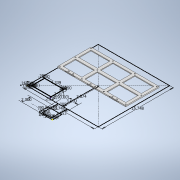
# Autodesk Inventor part: WellPlateFrame - 3L - Part1
Saved by Autodesk Inventor 2020 (Build 240168000, 168)
## iProperties
Created: 2023-02-18
Part Number: WellPlateFrame - 3L - Part1
Material: Generic
Document SubType Name: Modeling
Designer: Beaucage
Density: 1 g/cm^3
Appearance: Default
Author: Beaucage
Autodesk Inventor part; units mm, degrees
ref_plane "YZ Plane" through (0, 0, 0) normal (1, 0, 0) x (0, 1, 0)
ref_plane "XZ Plane" through (0, 0, 0) normal (0, 1, 0) x (-1, 0, 0)
ref_plane "XY Plane" through (0, 0, 0) normal (0, 0, 1) x (1, 0, 0)
sketch "Sketch1" plane through (0, 0, 0) normal (0, 1, 0) x (-1, 0, 0)
  line L0 (0, 0) -> (76.2, 0)
  line L1 (76.2, 0) -> (76.2, -50.8)
  line L2 (76.2, -50.8) -> (0, -50.8)
  line L3 (0, -50.8) -> (0, 0)
  line L4 (38.1, 0) -> (38.1, -6.35)
  line L5 (38.1, -6.35) -> (12.7, -6.35)
  line L6 (38.1, -6.35) -> (63.5, -6.35)
  line L7 (38.1, -6.35) -> (63.5, -6.35) construction
  line L8 (63.5, -6.35) -> (63.5, -19.05)
  line L9 (12.7, -6.35) -> (12.7, -19.05)
  line L10 (63.5, -19.05) -> (63.5, -25.4)
  line L11 (12.7, -19.05) -> (12.7, -25.4)
  line L12 (63.5, -19.05) -> (63.5, -94.05)
  line L13 (63.5, -19.05) -> (138.5, -19.05) construction
  line L14 (12.7, -19.05) -> (12.7, -94.05)
  line L15 (63.5, -94.05) -> (38.1, -94.05)
  line L16 (38.1, -94.05) -> (38.1, -294.05)
  line L17 (38.1, -94.05) -> (238.1, -94.05) construction
  line L18 (238.1, -494.05) -> (-161.9, -494.05)
  line L19 (-161.9, -494.05) -> (-161.9, -94.05)
  line L20 (-161.9, -94.05) -> (238.1, -94.05)
  line L21 (238.1, -94.05) -> (238.1, -494.05)
  line L22 (238.1, -494.05) -> (-161.9, -94.05) construction
  line L23 (-161.9, -494.05) -> (238.1, -94.05) construction
  point P0 (63.5, -50.8)
  point P1 (12.7, -50.8)
  dimension "d0" = 76.2
  dimension "d1" = 50.8
  dimension "d2" = 6.35
  dimension "d3" = 25.4
  dimension "d4" = 25.4
  dimension "d5" = 0
  dimension "d6" = 12.7
  dimension "d7" = 12.7
  dimension "d8" = 6.35
  dimension "d9" = 6.35
  dimension "d10" = 75
  dimension "d11" = 90
  dimension "d12" = 75
  dimension "d13" = 25.4
  dimension "d14" = 200
  dimension "d15" = 90
  dimension "d16" = 400
  dimension "d17" = 400
  constraints: 48 end point, 7 horizontal, 6 vertical, 4 parallel, 4 perpendicular, 3 equal length, 3 midpoint, 1 point on line
  measures "d0" distance of L1.end L2.end
  measures "d1" distance of L0.end L1.end
  measures "d2" distance of L4.start L4.end
  measures "d3" distance of L4.end L5.end
  measures "d4" distance of L4.end L6.end
  measures "d5" distance between parallel lines of L6 L7
  measures "d6" distance of L6.end L8.end
  measures "d7" distance of L5.end L9.end
  measures "d8" distance of L8.end L10.end
  measures "d9" distance of L9.end L11.end
  measures "d10" distance of L8.end L12.end
  measures "d11" angle of L12 L13
  measures "d12" distance of L9.end L14.end
  measures "d13" distance of L12.end L15.end
  measures "d14" distance of L15.end L16.end
  measures "d15" angle of L16 L17
  measures "d16" distance of L19.end L20.end
  measures "d17" distance of L18.end L19.end
extrude "Extrusion1" add sketch "Sketch1" along normal blind 6.35
hole "Hole1" at (-12.7, 0, -6.35) at (-12.7, 0, -19.05) at (-63.5, 0, -6.35) at (-63.5, 0, -19.05) direction (0, 1, 0) diameter 6.604 end through all
sketch "Sketch2" plane through (0, 0, 0) normal (0, -1, 0) x (1, 0, 0)
  line L0 (-238.1, -94.05) -> (-63.5, -94.05) projected
  line L1 (-238.1, -94.05) -> (-238.1, -100.4)
  line L2 (-238.1, -94.05) -> (-231.75, -94.05) construction
  line L3 (-238.1, -100.4) -> (-231.75, -100.4)
  line L4 (-231.75, -100.4) -> (-225.4, -100.4)
  line L5 (-225.4, -100.4) -> (-225.4, -106.75)
  line L6 (-225.4, -106.75) -> (-115.2, -106.75)
  line L7 (-115.2, -106.75) -> (-115.2, -180.75)
  line L8 (-115.2, -180.75) -> (-225.4, -180.75)
  line L9 (-225.4, -180.75) -> (-225.4, -106.75)
  line L10 (-115.2, -106.75) -> (-115.2, -100.4)
  line L11 (-115.2, -100.4) -> (-108.85, -100.4)
  line L12 (-225.4, -180.75) -> (-231.75, -180.75)
  line L13 (-231.75, -180.75) -> (-231.75, -187.1)
  line L14 (-115.2, -180.75) -> (-115.2, -187.1)
  line L15 (-115.2, -187.1) -> (-108.85, -187.1)
  line L16 (-225.4, -106.75) -> (-225.4, -114.75)
  line L17 (-225.4, -106.75) -> (-217.4, -106.75) construction
  line L18 (-225.4, -106.75) -> (-223.4, -106.75)
  line L19 (-223.4, -106.75) -> (-223.4, -108.75)
  line L20 (-223.4, -108.75) -> (-225.4, -108.75)
  line L21 (-225.4, -108.75) -> (-225.4, -106.75)
  line L22 (-115.2, -180.75) -> (-117.2, -180.75)
  line L23 (-117.2, -180.75) -> (-117.2, -178.75)
  line L24 (-117.2, -178.75) -> (-115.2, -178.75)
  line L25 (-115.2, -178.75) -> (-115.2, -180.75)
  line L26 (-223.4, -108.75) -> (-117.2, -108.75)
  line L27 (-117.2, -108.75) -> (-117.2, -178.75)
  line L28 (-117.2, -178.75) -> (-223.4, -178.75)
  line L29 (-223.4, -178.75) -> (-223.4, -108.75)
  point P0 (0, 0)
  dimension "d27" = 6.35
  dimension "d28" = 90
  dimension "d29" = 6.35
  dimension "d30" = 6.35
  dimension "d31" = 6.35
  dimension "d32" = 110.2
  dimension "d33" = 74
  dimension "d34" = 6.35
  dimension "d35" = 6.35
  dimension "d36" = 6.35
  dimension "d37" = 6.35
  dimension "d38" = 6.35
  dimension "d39" = 8
  dimension "d40" = 90
  dimension "d41" = 2
  dimension "d42" = 2
  dimension "d43" = 2
  dimension "d44" = 2
  constraints: 58 end point, 11 perpendicular, 8 horizontal, 8 parallel, 4 vertical
  measures "d27" distance of L0.start L1.end
  measures "d28" angle of L1 L2
  measures "d29" distance of L1.end L3.end
  measures "d30" distance of L3.end L4.end
  measures "d31" distance of L4.end L5.end
  measures "d32" distance of L7.end L8.end
  measures "d33" distance of L6.end L7.end
  measures "d34" distance of L10.end L11.end
  measures "d35" distance of L8.end L12.end
  measures "d36" distance of L12.end L13.end
  measures "d37" distance of L7.end L14.end
  measures "d38" distance of L14.end L15.end
  measures "d39" distance of L5.end L16.end
  measures "d40" angle of L16 L17
  measures "d41" distance of L19.end L20.end
  measures "d42" distance of L18.end L19.end
  measures "d43" distance of L23.end L24.end
  measures "d44" distance of L22.end L23.end
extrude "Extrusion2" cut sketch "Sketch2" against normal through all contours L26 L27 L28 L29
hole "Hole2" at (-231.75, 0, -100.4) at (-231.75, 0, -187.1) at (-108.85, 0, -100.4) at (-108.85, 0, -187.1) direction (0, 1, 0) diameter 5.1562 end through all
extrude "Extrusion3" cut sketch "Sketch2" against normal blind 2 contours L6 L19 L20 L9 | L6 L7 L24 L27 L26 L19 | L20 L29 L28 L23 L8 L9 | L7 L8 L23 L24
pattern_linear "Rectangular Pattern1" count 3 spacing 122.9106 along (1, 0, 0) count 4 spacing 86.9442 along (0, 0, -1) of "Extrusion2", "Hole2", "Extrusion3"
sketch "Sketch3" plane through (0, 0, 0) normal (0, -1, 0) x (1, 0, 0)
  circle A0 centre (136.9712, -447.9326) radius 2.5781 projected
  line L0 (136.9712, -447.9326) -> (143.3212, -447.9326)
  line L1 (143.3212, -447.9326) -> (143.3212, -454.2826)
  line L2 (143.3212, -454.2826) -> (136.9712, -454.2826)
  line L3 (136.9712, -454.2826) -> (136.9712, -447.9326)
  line L4 (-12.7, -94.05) -> (161.9, -94.05) projected
  line L5 (143.3212, -454.2826) -> (161.9, -454.2826)
  line L6 (161.9, -454.2826) -> (161.9, -94.05)
  line L7 (161.9, -94.05) -> (143.3212, -94.05)
  line L8 (143.3212, -94.05) -> (143.3212, -454.2826)
  line L9 (161.9, -454.2826) -> (-238.1, -454.2826)
  line L10 (-238.1, -454.2826) -> (-238.1, -500.3541)
  line L11 (-238.1, -500.3541) -> (161.9, -500.3541)
  line L12 (161.9, -500.3541) -> (161.9, -454.2826)
  point P0 (0, 0)
  dimension "d62" = 6.35
  dimension "d63" = 6.35
  constraints: 24 end point, 6 parallel, 3 horizontal, 3 perpendicular
  measures "d62" distance of L1.end L2.end
  measures "d63" distance of L0.end L1.end
extrude "Extrusion4" cut sketch "Sketch3" against normal through all contours L8 L4 L6 L5 L1 | L2 L5 L12 L11 L10 L9
sketch "Sketch4" plane through (0, 6.35, 0) normal (0, 1, 0) x (1, 0, 0)
  line L0 (-238.1, 454.2826) -> (-238.1, 94.05) projected
  line L1 (143.3212, 94.05) -> (143.3212, 454.2826) projected
  line L2 (-238.1, 454.2826) -> (143.3212, 454.2826)
  line L3 (143.3212, 454.2826) -> (143.3212, 265.3699)
  line L4 (143.3212, 265.3699) -> (-238.1, 265.3699)
  line L5 (-238.1, 265.3699) -> (-238.1, 454.2826)
  line L6 (143.3212, 265.3699) -> (-238.1, 265.3699)
  line L7 (-238.1, 265.3699) -> (-238.1, 0)
  line L8 (-238.1, 0) -> (143.3212, 0)
  line L9 (143.3212, 0) -> (143.3212, 265.3699)
  line L10 (-223.1708, 265.3699) -> (-238.1, 265.3699)
  line L11 (-117.2, 265.6942) -> (-223.4, 265.6942) projected
  line L12 (-223.4, 265.6942) -> (-238.1, 265.6942)
  line L13 (-238.1, 265.6942) -> (143.3212, 265.6942)
  line L14 (143.3212, 265.6942) -> (143.3212, 0)
  line L15 (143.3212, 0) -> (-238.1, 0)
  line L16 (-238.1, 0) -> (-238.1, 265.6942)
  line L17 (-225.4, 267.6942) -> (-238.1, 267.6942)
  line L18 (-238.1, 454.2826) -> (-238.1, 94.05) projected
  line L19 (-238.1, 267.6942) -> (143.3212, 267.6942)
  line L20 (143.3212, 267.6942) -> (143.3212, 0)
  line L21 (143.3212, 0) -> (-238.1, 0)
  line L22 (-238.1, 0) -> (-238.1, 267.6942)
  point P0 (0, 0)
  point P1 (143.3212, 265.6942)
  point P2 (143.3212, 267.6942)
  constraints: 38 end point, 8 parallel, 5 horizontal, 5 perpendicular, 5 point on line, 1 collinear
extrude "Extrusion5" cut sketch "Sketch4" against normal blind 25.4 contours L17 L19 L1 L13 L11 L12 L0 | L12 L11 L13 L1 L4 L0 | L4 L1 L9 L8 L7 L0
sketch "Sketch5" plane through (-238.1, 0, -267.6942) normal (0, 0, 1) x (1, 0, 0)
  line L0 (120.9, 2) -> (14.7, 2) projected
  line L1 (243.8106, 2) -> (137.6106, 2) projected
  line L2 (366.7212, 2) -> (260.5212, 2) projected
  line L3 (120.9, 6.35) -> (14.7, 6.35) projected
  line L4 (67.8, 6.35) -> (67.8, 3.175)
  line L5 (42.4, 4.7625) -> (93.2, 4.7625)
  line L6 (93.2, 4.7625) -> (93.2, 1.5875)
  line L7 (93.2, 1.5875) -> (42.4, 1.5875)
  line L8 (42.4, 1.5875) -> (42.4, 4.7625)
  line L9 (42.4, 4.7625) -> (93.2, 1.5875) construction
  line L10 (93.2, 4.7625) -> (42.4, 1.5875) construction
  line L11 (381.4212, 6.35) -> (0, 6.35) projected
  line L12 (190.7106, 6.35) -> (190.7106, 3.175)
  line L13 (165.3106, 1.5875) -> (216.1106, 1.5875)
  line L14 (216.1106, 1.5875) -> (216.1106, 4.7625)
  line L15 (216.1106, 4.7625) -> (165.3106, 4.7625)
  line L16 (165.3106, 4.7625) -> (165.3106, 1.5875)
  line L17 (165.3106, 1.5875) -> (216.1106, 4.7625) construction
  line L18 (216.1106, 1.5875) -> (165.3106, 4.7625) construction
  line L19 (260.5212, 6.35) -> (366.7212, 6.35) projected
  line L20 (313.6212, 6.35) -> (313.6212, 3.175)
  line L21 (288.2212, 1.5875) -> (339.0212, 1.5875)
  line L22 (339.0212, 1.5875) -> (339.0212, 4.7625)
  line L23 (339.0212, 4.7625) -> (288.2212, 4.7625)
  line L24 (288.2212, 4.7625) -> (288.2212, 1.5875)
  line L25 (288.2212, 1.5875) -> (339.0212, 4.7625) construction
  line L26 (339.0212, 1.5875) -> (288.2212, 4.7625) construction
  point P0 (238.1, 0)
  dimension "d68" = 3.175
  dimension "d69" = 50.8
  dimension "d70" = 3.175
  dimension "d71" = 50.8
  dimension "d72" = 3.175
  dimension "d73" = 3.175
  dimension "d74" = 50.8
  constraints: 42 end point, 9 midpoint, 6 parallel, 3 horizontal, 3 perpendicular, 3 vertical
  measures "d68" distance of L4.start L4.end
  measures "d69" distance of L6.end L7.end
  measures "d70" distance of L5.end L6.end
  measures "d71" distance of L15.end L14.end
  measures "d72" distance of L14.end L13.end
  measures "d73" distance of L20.start L20.end
  measures "d74" distance of L23.end L22.end
extrude "Extrusion6" cut sketch "Sketch5" against normal blind 3.175
sketch "Sketch6" plane through (0, 6.35, 0) normal (0, 1, 0) x (1, 0, 0)
  line L0 (-195.7, 267.6942) -> (-144.9, 267.6942) projected
  line L1 (-72.7894, 267.6942) -> (-21.9894, 267.6942) projected
  line L2 (50.1212, 267.6942) -> (100.9212, 267.6942) projected
  line L3 (-170.3, 267.6942) -> (-170.3, 274.0442)
  line L4 (-170.3, 274.0442) -> (-157.6, 274.0442)
  line L5 (-157.6, 274.0442) -> (-183, 274.0442)
  line L6 (-238.1, 267.6942) -> (143.3212, 267.6942) projected
  line L7 (-47.3894, 267.6942) -> (-47.3894, 274.0442)
  line L8 (-47.3894, 274.0442) -> (-34.6894, 274.0442)
  line L9 (-34.6894, 274.0442) -> (-60.0894, 274.0442)
  line L10 (50.1212, 267.6942) -> (75.5212, 267.6942)
  line L11 (75.5212, 267.6942) -> (75.5212, 274.0442)
  line L12 (75.5212, 274.0442) -> (88.2212, 274.0442)
  line L13 (88.2212, 274.0442) -> (62.8212, 274.0442)
  point P0 (0, 0)
  dimension "d77" = 6.35
  dimension "d78" = 12.7
  dimension "d79" = 25.4
  dimension "d80" = 12.7
  dimension "d81" = 25.4
  dimension "d82" = 25.4
  dimension "d83" = 6.35
  dimension "d84" = 12.7
  dimension "d85" = 90
  constraints: 20 end point, 4 perpendicular, 3 point on line, 2 vertical, 1 midpoint, 3 other
  measures "d77" distance of L3.start L3.end
  measures "d78" distance of L3.end L4.end
  measures "d79" distance of L4.end L5.end
  measures "d80" distance of L7.end L8.end
  measures "d81" distance of L8.end L9.end
  measures "d82" distance of L2.start L10.end
  measures "d83" distance of L10.end L11.end
  measures "d84" distance of L11.end L12.end
  measures "d85" angle of L11 L12
hole "Hole3" at (88.2212, 6.35, -274.0442) at (62.8212, 6.35, -274.0442) at (-34.6894, 6.35, -274.0442) at (-60.0894, 6.35, -274.0442) at (-183, 6.35, -274.0442) at (-157.6, 6.35, -274.0442) direction (0, -1, 0) diameter 6.7564 end through all clearance for "Socket Head Cap Screw" size "1/4" standard "Ansi Unified Screw Threads"
body "Solid1"
